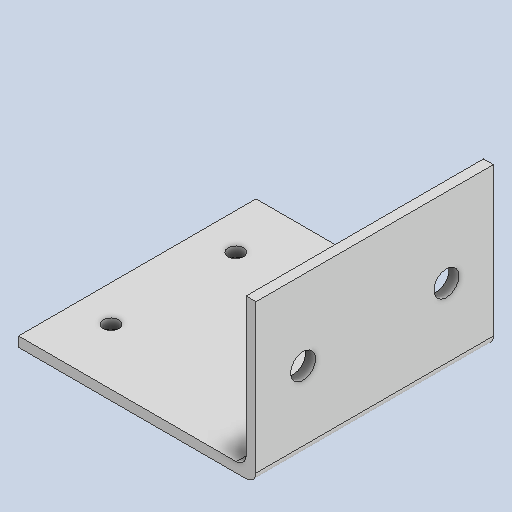
# Autodesk Inventor part: 2x3_L_Bracket
Saved by Autodesk Inventor 2023 (Build 270158000, 158)
## iProperties
Created: 2022-05-07
Part Number: 2x3_L_Bracket
Material: Generic
Document SubType Name: Modeling
Designer: plebbb
Density: 1 g/cm^3
Appearance: Default
Author: plebbb
Autodesk Inventor part; units mm, degrees
ref_plane "YZ Plane" through (0, 0, 0) normal (1, 0, 0) x (0, 1, 0)
ref_plane "XZ Plane" through (0, 0, 0) normal (0, 1, 0) x (-1, 0, 0)
ref_plane "XY Plane" through (0, 0, 0) normal (0, 0, 1) x (1, 0, 0)
sketch "Sketch1" plane through (0, 0, 0) normal (0, 0, 1) x (1, 0, 0)
  line L0 (0, 0) -> (76.2, 0)
  line L1 (76.2, 0) -> (76.2, 50.8)
  line L2 (76.2, 50.8) -> (0, 50.8)
  line L3 (0, 50.8) -> (0, 0)
  dimension "d0" = 76.2
  dimension "d1" = 50.8
  constraints: 8 end point, 3 perpendicular, 1 horizontal
  measures "d0" distance of L1.end L2.end
  measures "d1" distance of L0.end L1.end
extrude "Extrusion1" add sketch "Sketch1" along normal blind 76.2
shell "Shell1" thickness 3.175 removed faces 4 at (50.8, 16.9333, 76.2) at (50.8, 50.8, 25.4) at (50.8, 16.9333, 0) at (0, 33.8667, 25.4)
sketch "Sketch3" plane through (0, 0, 0) normal (0, -1, 0) x (1, 0, 0)
  line L0 (64.6, 58.1) -> (11.6, 58.1) construction
  line L1 (11.6, 58.1) -> (11.6, 18.1) construction
  line L2 (11.6, 18.1) -> (64.6, 18.1) construction
  line L3 (64.6, 18.1) -> (64.6, 58.1) construction
  circle A0 centre (64.6, 18.1) radius 2.5
  circle A1 centre (64.6, 58.1) radius 2.5
  circle A2 centre (11.6, 58.1) radius 2.5
  circle A3 centre (11.6, 18.1) radius 2.5
  line L4 (76.2, 0) -> (76.2, 76.2) construction
  line L5 (0, 76.2) -> (76.2, 76.2) construction
  point P0 (0, 0)
  point P1 (64.6, 38.1)
  point P2 (76.2, 38.1)
  point P3 (38.1, 58.1)
  point P4 (38.1, 76.2)
  dimension "d6" = 40
  dimension "d7" = 53
  dimension "d8" = 5
  constraints: 8 end point, 4 centre point, 4 coincident, 4 midpoint, 3 equal radius, 2 parallel, 1 horizontal, 1 horizontal alignment, 1 perpendicular, 1 vertical alignment
  measures "d6" distance of L2.end L0.start
  measures "d7" distance of L1.end L2.end
  measures "d8" diameter of A1
extrude "Extrusion2" cut sketch "Sketch3" against normal blind 76.2
sketch "Sketch4" plane through (76.2, 0, 0) normal (1, 0, 0) x (0, 0, -1)
  circle A0 centre (-61.1, 25.4) radius 4
  circle A1 centre (-15.1, 25.4) radius 4
  line L0 (-61.1, 25.4) -> (-15.1, 25.4) construction
  line L1 (0, 0) -> (0, 50.8) construction
  line L2 (0, 50.8) -> (-76.2, 50.8) construction
  line L3 (-76.2, 0) -> (-76.2, 50.8) construction
  line L4 (0, 0) -> (-76.2, 0) construction
  point P0 (-38.1, 25.4)
  point P1 (0, 25.4)
  point P2 (-38.1, 50.8)
  dimension "d11" = 46
  dimension "d12" = 8
  constraints: 3 midpoint, 2 centre point, 2 end point, 1 coincident, 1 equal radius, 1 horizontal, 1 horizontal alignment, 1 vertical alignment
  measures "d11" distance of L0.start L0.end
  measures "d12" diameter of A0
extrude "Extrusion3" cut sketch "Sketch4" against normal blind 76.2
fillet "Fillet1" radius 3.175 2 edges at (76.2, 0, 38.1) (73.025, 3.175, 38.1)
body "Solid1"
